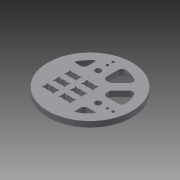
# Autodesk Inventor part: Segment
Saved by Autodesk Inventor 2015 (Build 190159000, 159)
## iProperties
Created: 2012-09-02
Part Number: Segment
Material: Generic
Document SubType Name: Modeling
Designer: ErikEnvy
Density: 1 g/cm^3
Appearance: Default
Author: ErikEnvy
Autodesk Inventor part; units mm, degrees
ref_plane "YZ Plane" through (0, 0, 0) normal (1, 0, 0) x (0, 1, 0)
ref_plane "XZ Plane" through (0, 0, 0) normal (0, 1, 0) x (-1, 0, 0)
ref_plane "XY Plane" through (0, 0, 0) normal (0, 0, 1) x (1, 0, 0)
sketch "Sketch1" plane through (0, 0, 0) normal (0, 0, 1) x (1, 0, 0)
  circle A0 centre (0, 15) radius 1.6
  circle A1 centre (15, 0) radius 1.6
  circle A2 centre (5.3033, 5.3033) radius 22.5
  circle A3 centre (0, 20) radius 0.75
  circle A4 centre (20, 0) radius 0.75
  circle A5 centre (23, 0) radius 0.75
  circle A6 centre (0, 23) radius 0.75
  line L0 (5, 20.7102) -> (5, 14.5)
  line L1 (-5, 18.4292) -> (-5, 14.5)
  line L2 (20.7102, 5) -> (14.5, 5)
  line L3 (18.4292, -5) -> (14.5, -5)
  line L4 (9.5503, 13.0858) -> (14.0236, 17.5592)
  line L5 (13.0858, 9.5503) -> (17.5592, 14.0236)
  arc A7 (-5.8177, 18.8152) -> (-10.3004, 13.2264) centre (5.3033, 5.3033) ccw
  line L6 (8.136, 12.5) -> (7, 12.5)
  line L7 (-7, 12.5) -> (-9.8546, 12.5)
  line L8 (12.5, -9.8546) -> (12.5, -7)
  line L9 (12.5, 7) -> (12.5, 8.136)
  arc A8 (13.2264, -10.3004) -> (18.8152, -5.8177) centre (5.3033, 5.3033) ccw
  arc A9 (22.6981, 7.2189) -> (20.7372, 13.5521) centre (5.3033, 5.3033) ccw
  arc A10 (13.5521, 20.7372) -> (7.2189, 22.6981) centre (5.3033, 5.3033) ccw
  arc A11 (7.2189, 22.6981) -> (5, 20.7102) centre (7, 20.7102) ccw
  arc A12 (14.0236, 17.5592) -> (13.5521, 20.7372) centre (12.6094, 18.9734) ccw
  arc A13 (5, 14.5) -> (7, 12.5) centre (7, 14.5) ccw
  arc A14 (8.136, 12.5) -> (9.5503, 13.0858) centre (8.136, 14.5) ccw
  arc A15 (13.0858, 9.5503) -> (12.5, 8.136) centre (14.5, 8.136) ccw
  arc A16 (12.5, 7) -> (14.5, 5) centre (14.5, 7) ccw
  arc A17 (20.7102, 5) -> (22.6981, 7.2189) centre (20.7102, 7) ccw
  arc A18 (20.7372, 13.5521) -> (17.5592, 14.0236) centre (18.9734, 12.6094) ccw
  arc A19 (-7, 12.5) -> (-5, 14.5) centre (-7, 14.5) ccw
  arc A20 (14.5, -5) -> (12.5, -7) centre (14.5, -7) ccw
  arc A21 (18.8152, -5.8177) -> (18.4292, -5) centre (18.4292, -5.5) ccw
  arc A22 (12.5, -9.8546) -> (13.2264, -10.3004) centre (13, -9.8546) ccw
  arc A23 (-10.3004, 13.2264) -> (-9.8546, 12.5) centre (-9.8546, 13) ccw
  arc A24 (-5, 18.4292) -> (-5.8177, 18.8152) centre (-5.5, 18.4292) ccw
  arc A25 (-7.25, 7.5) -> (-7.5, 7.25) centre (-7.5, 7.5) ccw
  arc A26 (-6.75, 7.5) -> (-5.25, 7.5) centre (-6, 8.8062) ccw
  arc A27 (-1.5, 7.25) -> (-1.75, 7.5) centre (-1.5, 7.5) ccw
  arc A28 (-3.75, 7.5) -> (-2.25, 7.5) centre (-3, 8.8062) ccw
  arc A29 (-7.5, 4.75) -> (-7.25, 4.5) centre (-7.5, 4.5) ccw
  arc A30 (-5.25, 4.5) -> (-6.75, 4.5) centre (-6, 3.1938) ccw
  arc A31 (-2.25, 4.5) -> (-3.75, 4.5) centre (-3, 3.1938) ccw
  arc A32 (-1.75, 4.5) -> (-1.5, 4.75) centre (-1.5, 4.5) ccw
  line L10 (-1.5, 7.25) -> (-1.5, 4.75)
  line L11 (-1.75, 4.5) -> (-2.25, 4.5)
  line L12 (-2.25, 7.5) -> (-1.75, 7.5)
  line L13 (-3.75, 7.5) -> (-5.25, 7.5)
  line L14 (-5.25, 4.5) -> (-3.75, 4.5)
  line L15 (-7.25, 7.5) -> (-6.75, 7.5)
  line L16 (-7.5, 7.25) -> (-7.5, 4.75)
  line L17 (-6.75, 4.5) -> (-7.25, 4.5)
  arc A33 (1.75, 7.5) -> (1.5, 7.25) centre (1.5, 7.5) ccw
  arc A34 (2.25, 7.5) -> (3.75, 7.5) centre (3, 8.8062) ccw
  arc A35 (5.25, 7.5) -> (6.75, 7.5) centre (6, 8.8062) ccw
  arc A36 (7.5, 7.25) -> (7.25, 7.5) centre (7.5, 7.5) ccw
  arc A37 (6.75, 4.5) -> (5.25, 4.5) centre (6, 3.1938) ccw
  arc A38 (7.25, 4.5) -> (7.5, 4.75) centre (7.5, 4.5) ccw
  arc A39 (3.75, 4.5) -> (2.25, 4.5) centre (3, 3.1938) ccw
  arc A40 (1.5, 4.75) -> (1.75, 4.5) centre (1.5, 4.5) ccw
  line L18 (7.5, 7.25) -> (7.5, 4.75)
  line L19 (7.25, 4.5) -> (6.75, 4.5)
  line L20 (6.75, 7.5) -> (7.25, 7.5)
  line L21 (5.25, 7.5) -> (3.75, 7.5)
  line L22 (3.75, 4.5) -> (5.25, 4.5)
  line L23 (1.75, 7.5) -> (2.25, 7.5)
  line L24 (1.5, 7.25) -> (1.5, 4.75)
  line L25 (2.25, 4.5) -> (1.75, 4.5)
  arc A41 (-7.25, 1.5) -> (-7.5, 1.25) centre (-7.5, 1.5) ccw
  arc A42 (-6.75, 1.5) -> (-5.25, 1.5) centre (-6, 2.8062) ccw
  arc A43 (-3.75, 1.5) -> (-2.25, 1.5) centre (-3, 2.8062) ccw
  arc A44 (-1.5, 1.25) -> (-1.75, 1.5) centre (-1.5, 1.5) ccw
  arc A45 (-2.25, -1.5) -> (-3.75, -1.5) centre (-3, -2.8062) ccw
  arc A46 (-1.75, -1.5) -> (-1.5, -1.25) centre (-1.5, -1.5) ccw
  arc A47 (-5.25, -1.5) -> (-6.75, -1.5) centre (-6, -2.8062) ccw
  arc A48 (-7.5, -1.25) -> (-7.25, -1.5) centre (-7.5, -1.5) ccw
  line L26 (-1.5, 1.25) -> (-1.5, -1.25)
  line L27 (-1.75, -1.5) -> (-2.25, -1.5)
  line L28 (-2.25, 1.5) -> (-1.75, 1.5)
  line L29 (-3.75, 1.5) -> (-5.25, 1.5)
  line L30 (-5.25, -1.5) -> (-3.75, -1.5)
  line L31 (-7.25, 1.5) -> (-6.75, 1.5)
  line L32 (-7.5, 1.25) -> (-7.5, -1.25)
  line L33 (-6.75, -1.5) -> (-7.25, -1.5)
  arc A49 (1.75, 1.5) -> (1.5, 1.25) centre (1.5, 1.5) ccw
  arc A50 (2.25, 1.5) -> (3.75, 1.5) centre (3, 2.8062) ccw
  arc A51 (5.25, 1.5) -> (6.75, 1.5) centre (6, 2.8062) ccw
  arc A52 (7.5, 1.25) -> (7.25, 1.5) centre (7.5, 1.5) ccw
  arc A53 (6.75, -1.5) -> (5.25, -1.5) centre (6, -2.8062) ccw
  arc A54 (7.25, -1.5) -> (7.5, -1.25) centre (7.5, -1.5) ccw
  arc A55 (3.75, -1.5) -> (2.25, -1.5) centre (3, -2.8062) ccw
  arc A56 (1.5, -1.25) -> (1.75, -1.5) centre (1.5, -1.5) ccw
  line L34 (7.5, 1.25) -> (7.5, -1.25)
  line L35 (7.25, -1.5) -> (6.75, -1.5)
  line L36 (6.75, 1.5) -> (7.25, 1.5)
  line L37 (5.25, 1.5) -> (3.75, 1.5)
  line L38 (3.75, -1.5) -> (5.25, -1.5)
  line L39 (1.75, 1.5) -> (2.25, 1.5)
  line L40 (1.5, 1.25) -> (1.5, -1.25)
  line L41 (2.25, -1.5) -> (1.75, -1.5)
  arc A57 (-7.25, -4.5) -> (-7.5, -4.75) centre (-7.5, -4.5) ccw
  arc A58 (-6.75, -4.5) -> (-5.25, -4.5) centre (-6, -3.1938) ccw
  arc A59 (-3.75, -4.5) -> (-2.25, -4.5) centre (-3, -3.1938) ccw
  arc A60 (-1.5, -4.75) -> (-1.75, -4.5) centre (-1.5, -4.5) ccw
  arc A61 (-2.25, -7.5) -> (-3.75, -7.5) centre (-3, -8.8062) ccw
  arc A62 (-1.75, -7.5) -> (-1.5, -7.25) centre (-1.5, -7.5) ccw
  arc A63 (-5.25, -7.5) -> (-6.75, -7.5) centre (-6, -8.8062) ccw
  arc A64 (-7.5, -7.25) -> (-7.25, -7.5) centre (-7.5, -7.5) ccw
  line L42 (-1.5, -4.75) -> (-1.5, -7.25)
  line L43 (-1.75, -7.5) -> (-2.25, -7.5)
  line L44 (-2.25, -4.5) -> (-1.75, -4.5)
  line L45 (-3.75, -4.5) -> (-5.25, -4.5)
  line L46 (-5.25, -7.5) -> (-3.75, -7.5)
  line L47 (-7.25, -4.5) -> (-6.75, -4.5)
  line L48 (-7.5, -4.75) -> (-7.5, -7.25)
  line L49 (-6.75, -7.5) -> (-7.25, -7.5)
  arc A65 (1.75, -4.5) -> (1.5, -4.75) centre (1.5, -4.5) ccw
  arc A66 (2.25, -4.5) -> (3.75, -4.5) centre (3, -3.1938) ccw
  arc A67 (5.25, -4.5) -> (6.75, -4.5) centre (6, -3.1938) ccw
  arc A68 (7.5, -4.75) -> (7.25, -4.5) centre (7.5, -4.5) ccw
  arc A69 (6.75, -7.5) -> (5.25, -7.5) centre (6, -8.8062) ccw
  arc A70 (7.25, -7.5) -> (7.5, -7.25) centre (7.5, -7.5) ccw
  arc A71 (3.75, -7.5) -> (2.25, -7.5) centre (3, -8.8062) ccw
  arc A72 (1.5, -7.25) -> (1.75, -7.5) centre (1.5, -7.5) ccw
  line L50 (7.5, -4.75) -> (7.5, -7.25)
  line L51 (7.25, -7.5) -> (6.75, -7.5)
  line L52 (6.75, -4.5) -> (7.25, -4.5)
  line L53 (5.25, -4.5) -> (3.75, -4.5)
  line L54 (3.75, -7.5) -> (5.25, -7.5)
  line L55 (1.75, -4.5) -> (2.25, -4.5)
  line L56 (1.5, -4.75) -> (1.5, -7.25)
  line L57 (2.25, -7.5) -> (1.75, -7.5)
  point P0 (-10.6484, 12.5)
  point P1 (19.3185, 15.783)
  point P2 (12.5, -10.6484)
  point P3 (-5, 19.4487)
  point P4 (19.4487, -5)
  point P5 (22.8007, 5)
  point P6 (15.783, 19.3185)
  point P7 (5, 22.8007)
  constraints: 140 point on circle, 116 end point, 73 centre point, 28 tangent, 11 equal radius, 11 perpendicular, 8 point on line, 4 parallel, 1 coincident, 1 collinear
extrude "Extrusion1" add sketch "Sketch1" along normal blind 3
body "Solid1"
